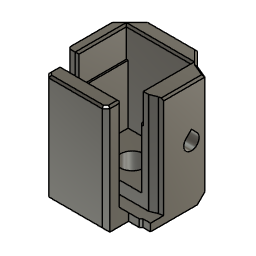
Ethernet_HAT_holder (Autodesk Fusion 360 design; units mm, degrees)
Autodesk Fusion 360 part; units mm, degrees
sketch "Sketch1" plane through (0, 0, 0) normal (0, 0, 1) x (1, 0, 0)
  line L0 (0, 0) -> (23, 0)
  line L1 (23, 0) -> (23, 17)
  line L2 (23, 17) -> (0, 17)
  line L3 (0, 17) -> (0, 0)
  dimension "d1" = 23
  dimension "d2" = 17
  constraint horizontal L0
  constraint vertical L1
  constraint horizontal L2
  constraint vertical L3
  constraint coincident L0.start L3.end
  measures "d1" distance of L1.end L2.end
  measures "d2" distance of L0.end L1.end
extrude "Extrude1" add sketch "Sketch1" along normal blind 28
sketch "Sketch2" plane through (0, 0, 28) normal (0, 0, 1) x (-1, 0, 0)
  line L0 (0, -17) -> (0, 0)
  line L1 (0, 0) -> (-23, 0)
  line L2 (-23, 0) -> (-23, -17)
  line L3 (-23, -17) -> (0, -17)
  line L4 (-3.36, 0) -> (-19.64, 0)
  line L5 (-19.64, 0) -> (-19.64, -13.15)
  line L6 (-3.36, -13.15) -> (-3.36, 0)
  line L7 (-3.36, -13.15) -> (-11.5, -13.15)
  line L8 (-11.5, -13.15) -> (-19.64, -13.15)
  dimension "d5" = 16.28
  dimension "d6" = 8.14
  dimension "d7" = 11.5
  dimension "d8" = 23
  dimension "d9" = 13.15
  constraint horizontal L4
  constraint vertical L5
  constraint vertical L6
  constraint coincident L1 L4.start
  constraint perpendicular L5 L7
  constraint perpendicular L5 L8
  measures "d5" distance of L5.end L6.start
  measures "d6" distance of L5.end L7.end
  measures "d7" horizontal distance of L1.end L7.end
  measures "d8" distance of L0.start L2.end
  measures "d9" distance of L4.end L5.end
extrude "Extrude2" cut sketch "Sketch2" against normal blind 23.68 contours L1 L4 L5 L6 L7 L8
sketch "Sketch3" plane through (0, 0, 28) normal (0, 0, 1) x (-1, 0, 0)
  line L0 (-3.36, 0) -> (-3.36, -13.15)
  line L1 (-3.36, -13.15) -> (-19.64, -13.15)
  line L2 (-19.64, -13.15) -> (-19.64, 0)
  line L3 (-19.64, 0) -> (-23, 0)
  line L4 (-23, 0) -> (-23, -17)
  line L5 (-23, -17) -> (0, -17)
  line L6 (0, -17) -> (0, 0)
  line L7 (0, 0) -> (-3.36, 0)
  line L8 (0, 0) -> (-23, 0)
  line L9 (-23, 0) -> (-23, -3)
  line L10 (-23, -3) -> (0, -3)
  line L11 (0, -3) -> (0, 0)
  dimension "d12" = 3
  constraint horizontal L8
  constraint vertical L9
  constraint horizontal L10
  constraint vertical L11
  constraint coincident L6.end L7.start
  measures "d12" distance of L6.end L10.end
extrude "Extrude3" cut sketch "Sketch3" against normal blind 23.68 contours L0 L6 L7 L8 L10 L11 | L2 L3 L4 L8 L9 L10
sketch "Sketch4" plane through (23, 0, 0) normal (1, 0, 0) x (0, 1, 0)
  line L0 (3, 4.32) -> (0, 4.32)
  line L1 (0, 4.32) -> (0, 0)
  line L2 (0, 0) -> (17, 0)
  line L3 (17, 0) -> (17, 28)
  line L4 (17, 28) -> (3, 28)
  line L5 (3, 28) -> (3, 4.32)
  line L6 (3, 4.32) -> (3, 28)
  line L7 (3, 28) -> (13.15, 28)
  line L8 (13.15, 28) -> (13.15, 4.32)
  line L9 (13.15, 4.32) -> (3, 4.32)
  line L10 (6.9741, 15.7766) -> (8.4307, 17.2333)
  line L11 (8.4307, 17.2333) -> (9.8873, 15.7766)
  arc A0 (6.9741, 15.7766) -> (9.8873, 15.7766) centre (8.4307, 14.32) ccw
  line L12 (8.4307, 14.32) -> (11.5, 14.32)
  line L13 (8.4307, 14.32) -> (8.4307, 17.2333)
  dimension "d15" = 4.12
  dimension "d16" = 5.4307
  dimension "d17" = 10
  dimension "d18" = 90
  dimension "d57" = 90
  constraint tangent L10 A0
  constraint tangent L11 A0
  constraint coincident A0.centre L12.start
  constraint horizontal L12
  measures "d15" diameter of A0
  measures "d16" distance of L6 A0.centre
  measures "d17" distance of L9 A0.centre
  measures "d18" angle of L10 L11
  measures "d57" angle of L12 L13
extrude "Extrude4" cut sketch "Sketch4" against normal blind 10 contours L10 A0 L12 L13 | L11 A0 L12 L13
extrude "Extrude6" add 1 faces at (7.6667, 11.3333, 0) along direction (0, 0, -1) blind 11
sketch "Sketch7" plane through (0, 0, 28) normal (0, 0, 1) x (-1, 0, 0)
  line L0 (0, -3) -> (-3.36, -3)
  line L1 (-3.36, -3) -> (-3.36, -13.15)
  line L2 (-3.36, -13.15) -> (-19.64, -13.15)
  line L3 (-19.64, -13.15) -> (-19.64, -3)
  line L4 (-19.64, -3) -> (-23, -3)
  line L5 (-23, -3) -> (-23, -17)
  line L6 (-23, -17) -> (0, -17)
  line L7 (0, -17) -> (0, -3)
  line L8 (-2.9, -3) -> (-20.1, -3)
  line L9 (-20.1, -3) -> (-20.1, -13.15)
  line L10 (-2.9, -13.15) -> (-2.9, -3)
  line L11 (-2.9, -13.15) -> (-11.5, -13.15)
  line L12 (-11.5, -13.15) -> (-20.1, -13.15)
  point P0 (-23, 0)
  dimension "d33" = 17.2
  dimension "d34" = 8.6
  dimension "d35" = 11.5
  dimension "d36" = 23
  dimension "d37" = 10.15
  dimension "d38" = 10.15
  constraint horizontal L8
  constraint vertical L9
  constraint vertical L10
  constraint coincident L0 L8.start
  constraint perpendicular L9 L11
  constraint perpendicular L9 L12
  measures "d33" distance of L9.end L10.start
  measures "d34" distance of L10.start L11.end
  measures "d35" horizontal distance of L11.end P0
  measures "d36" distance of L5.end L6.end
  measures "d37" distance of L2.end L3.end
  measures "d38" distance of L8.end L9.end
extrude "Extrude8" cut sketch "Sketch7" against normal blind 8 contours L0 L1 L8 L10 L11 | L3 L4 L8 L9 L12
chamfer "Chamfer1" distance 5 angle 45 2 edges at (23, 17, 8.5) (0, 17, 8.5)
extrude "Extrude11" add 2 faces at (20.9133, 3, 9.5467) (2.0867, 3, 9.5467) along direction (0, -1, 0) blind 3
sketch "Sketch10" plane through (0, 0, 0) normal (0, -1, 0) x (1, 0, 0)
  line L0 (19.64, 4.32) -> (3.36, 4.32)
  line L1 (3.36, 4.32) -> (3.36, 20)
  line L2 (3.36, 20) -> (2.9, 20)
  line L3 (2.9, 20) -> (2.9, 28)
  line L4 (2.9, 28) -> (0, 28)
  line L5 (0, 28) -> (0, -11)
  line L6 (0, -11) -> (23, -11)
  line L7 (23, -11) -> (23, 28)
  line L8 (23, 28) -> (20.1, 28)
  line L9 (20.1, 28) -> (20.1, 20)
  line L10 (20.1, 20) -> (19.64, 20)
  line L11 (19.64, 20) -> (19.64, 4.32)
  line L12 (0, -11) -> (23, -11)
  line L13 (23, -11) -> (23, 1)
  line L14 (23, 1) -> (0, 1)
  line L15 (0, 1) -> (0, -11)
  dimension "d52" = 12
  constraint horizontal L12
  constraint vertical L13
  constraint horizontal L14
  constraint vertical L15
  constraint coincident L5.end L6.start
  measures "d52" distance of L5.end L14.end
extrude "Extrude12" add sketch "Sketch10" along normal blind 3 contours L5 L6 L7 L12 L13 L14 L15
extrude "Extrude13" cut 1 faces at (7.6667, 3, -11) along direction (0, 0, 1) blind 10
sketch "Sketch11" plane through (0, 0, -1) normal (0, 0, -1) x (1, 0, 0)
  line L0 (0, -12) -> (5, -17)
  line L1 (5, -17) -> (18, -17)
  line L2 (18, -17) -> (23, -12)
  line L3 (23, -12) -> (23, 3)
  line L4 (23, 3) -> (0, 3)
  line L5 (0, 3) -> (0, -12)
  line L6 (0, 3) -> (23, 3)
  line L7 (3.36, 0) -> (19.64, 0)
  line L8 (19.64, 0) -> (19.64, 15.1403)
  line L9 (19.64, 15.1403) -> (3.36, 15.1403)
  line L10 (3.36, 15.1403) -> (3.36, 0)
  line L11 (3.36, 3) -> (19.64, 3)
  line L12 (19.64, 3) -> (19.64, 9)
  line L13 (19.64, 9) -> (3.36, 9)
  line L14 (3.36, 9) -> (3.36, 3)
  point P0 (3.36, 0)
  point P1 (19.64, 0)
  dimension "d60" = 6
  constraint horizontal L7
  constraint vertical L8
  constraint horizontal L9
  constraint vertical L10
  constraint coincident P0 L7.start
  constraint horizontal L11
  constraint vertical L12
  constraint horizontal L13
  constraint vertical L14
  constraint coincident L6 L11.start
  constraint coincident L10 L11.start
  measures "d60" distance of L11.start L13.end
extrude "Extrude14" add sketch "Sketch11" against normal blind 29 contours L4 L6 L8 L10 L11 L12 L13 L14
ref_plane "WorkPlane1" through (11.5, 17, 28) normal (0, 0.707107, 0.707107) x (-1, 0, 0)
sketch "Sketch12" plane through (0, 22.5, 22.5) normal (0, 0.707107, 0.707107) x (-1, 0, 0)
  line L0 (-20.1, 10.5005) -> (-2.9, 10.5005)
  line L1 (-2.9, 10.5005) -> (-2.9, 4.8437)
  line L2 (-2.9, 4.8437) -> (-3.36, 4.8437)
  line L3 (-3.36, 4.8437) -> (-3.36, -6.2438)
  line L4 (-3.36, -6.2438) -> (-19.64, -6.2438)
  line L5 (-19.64, -6.2438) -> (-19.64, 4.8437)
  line L6 (-19.64, 4.8437) -> (-20.1, 4.8437)
  line L7 (-20.1, 4.8437) -> (-20.1, 10.5005)
  line L8 (-12.9849, -3.0145) -> (-11.5, -1.5296)
  line L9 (-11.5, -1.5296) -> (-10.0151, -3.0145)
  arc A0 (-12.9849, -3.0145) -> (-10.0151, -3.0145) centre (-11.5, -4.4995) ccw
  dimension "d64" = 4.2
  dimension "d65" = 15
  dimension "d70" = 90
  dimension "d71" = 8.14
  constraint vertical A0.centre L8.end
  constraint tangent L8 A0
  constraint tangent L9 A0
  measures "d64" diameter of A0
  measures "d65" distance of L0 A0.centre
  measures "d70" angle of L8 L9
  measures "d71" distance of L3 A0.centre
extrude "Extrude15" cut sketch "Sketch12" against normal blind 19.45 contours L4 L8 L9 A0 | L4 A0
chamfer "Chamfer4" distance 7 angle 45 1 edges at (11.5, 17, -1)
sketch "Sketch13" plane through (0, 0, 28) normal (0, 0, 1) x (-1, 0, 0)
  line L0 (-3.36, 3) -> (-3.36, 9)
  line L1 (-3.36, 9) -> (-19.64, 9)
  line L2 (-19.64, 9) -> (-19.64, 3)
  line L3 (-19.64, 3) -> (-3.36, 3)
  line L4 (-19.64, 3) -> (-3.36, 3)
  line L5 (-3.36, 3) -> (-3.36, 6)
  line L6 (-3.36, 6) -> (-19.64, 6)
  line L7 (-19.64, 6) -> (-19.64, 3)
  dimension "d72" = 3
  constraint horizontal L4
  constraint vertical L5
  constraint horizontal L6
  constraint vertical L7
  constraint coincident L2.end L3.start
  measures "d72" distance of L2.end L6.end
extrude "Extrude16" cut sketch "Sketch13" against normal blind 27 contours L0 L2 L3 L4 L5 L6 L7
chamfer "Chamfer7" distance 1 angle 45 4 edges at (23, 0, 14.5) (19.64, -9, 13.5) (0, 0, 14.5) (3.36, -9, 13.5)
chamfer "Chamfer9" distance 0.5 angle 45 2 edges at (23, -3, 0) (0, -3, 0)
chamfer "Chamfer14" distance 1 angle 45 1 edges at (11.5, -9, -1)
extrude "Extrude23" add 3 faces at (23, -0.8333, -0.3333) (23, 7.8102, 24.4111) (23, 2.3333, 20.1067) along direction (1, 0, 0) blind 2
chamfer "Chamfer15" distance 1.4 angle 45 1 edges at (23, 1, 14.5)
chamfer "Chamfer16" distance 2 angle 45 1 edges at (23, 12, 14.5)
chamfer "Chamfer17" distance 0.6 angle 45 1 edges at (24.4, 1, 14.5)
sketch "Sketch15" plane through (0, 0, 1) normal (0, 0, 1) x (-1, 0, 0)
  line L0 (-25, -1) -> (-23.8457, -0.7704)
  line L1 (-23.8457, -0.7704) -> (-22.0101, -0.0101)
  line L2 (-22.0101, -0.0101) -> (-22, 0)
  line L3 (-22, 0) -> (-1, 0)
  line L4 (-1, 0) -> (0, -1)
  line L5 (0, -1) -> (0, 2.5)
  line L6 (0, 2.5) -> (-0.5, 3)
  line L7 (-0.5, 3) -> (-3.36, 3)
  line L8 (-3.36, 3) -> (-3.36, 6)
  line L9 (-3.36, 6) -> (-19.64, 6)
  line L10 (-19.64, 6) -> (-19.64, 3)
  line L11 (-19.64, 3) -> (-22.5, 3)
  line L12 (-22.5, 3) -> (-23, 2.5)
  line L13 (-23, 2.5) -> (-25, 2.5)
  line L14 (-25, 2.5) -> (-25, -1)
  line L15 (-19.64, 6) -> (-3.36, 6)
  line L16 (-3.36, 6) -> (-3.36, 5)
  line L17 (-3.36, 5) -> (-19.64, 5)
  line L18 (-19.64, 5) -> (-19.64, 6)
  dimension "d102" = 1
  constraint horizontal L15
  constraint vertical L16
  constraint horizontal L17
  constraint vertical L18
  constraint coincident L9.end L10.start
  measures "d102" distance of L9.end L17.end
extrude "Extrude24" add sketch "Sketch15" along normal blind 27 contours L8 L9 L10 L15 L16 L17 L18
chamfer "Chamfer18" distance 2 angle 45 1 edges at (11.5, -5, 1)
chamfer "Chamfer19" distance 0.5 angle 45 6 edges at (19.64, -5, 15.5) (3.36, -5, 15.5) (2.9, 0, 24) (3.36, 0, 12.16) (19.64, 0, 12.16) (20.1, 0, 24)
chamfer "Chamfer20" distance 0.5 angle 45 4 edges at (11.5, -5, 28) (2.9, 6.825, 28) (11.5, 13.15, 28) (20.1, 6.825, 28)
sketch "Sketch16" plane through (0, 0, 4.32) normal (0, 0, 1) x (-1, 0, 0)
  line L0 (-2.86, 0) -> (-20.14, 0)
  line L1 (-20.14, 0) -> (-19.64, -0.5)
  line L2 (-19.64, -0.5) -> (-19.64, -13.15)
  line L3 (-19.64, -13.15) -> (-3.36, -13.15)
  line L4 (-3.36, -13.15) -> (-3.36, -0.5)
  line L5 (-3.36, -0.5) -> (-2.86, 0)
  circle A0 centre (-11.5, -6.15) radius 3.25
  dimension "d108" = 6.5
  dimension "d111" = 7
  measures "d108" diameter of A0
  measures "d111" distance of L3 A0.centre
extrude "Extrude25" cut sketch "Sketch16" against normal blind 5.32 contours A0
chamfer "Chamfer22" distance 0.5 angle 45 6 edges at (11.5, 17, 28) (25, 6.5, 28) (23.2929, 12.7071, 28) (19.7929, 15.2071, 28) (2.5, 14.5, 28) (0, 6.5, 28)
chamfer "Chamfer23" distance 0.5 angle 45 5 edges at (11.5, -9, 28) (3.86, -8.5, 28) (3.36, -6.75, 28) (19.14, -8.5, 28) (19.64, -6.75, 28)
equation "d5 = 16.13 mm + 0.15 mm"
equation "d6 = d5 / 2"
equation "d7 = d8 / 2"
equation "d10 = -23.53 mm - 0.15 mm"
equation "d34 = d33 / 2"
equation "d35 = d36 / 2"
equation "d38 = d37"
